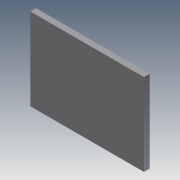
# Autodesk Inventor part: backbase
Saved by Autodesk Inventor 2011 (Build 150239000, 239)
## iProperties
Created: 2011-12-10
Part Number: backbase
Document SubType Name: Modeling
Designer: Matthew
Density: 1 g/cm^3
Author: Matthew
Autodesk Inventor part; units mm, degrees
ref_plane "YZ Plane" through (0, 0, 0) normal (1, 0, 0) x (0, 1, 0)
ref_plane "XZ Plane" through (0, 0, 0) normal (0, 1, 0) x (-1, 0, 0)
ref_plane "XY Plane" through (0, 0, 0) normal (0, 0, 1) x (1, 0, 0)
sketch "Sketch1" plane through (0, 0, 0) normal (0, 0, 1) x (1, 0, 0)
  line L0 (-30.3426, 15.2936) -> (25.6574, 15.2936)
  line L1 (25.6574, 15.2936) -> (25.6574, -29.7064)
  line L2 (25.6574, -29.7064) -> (-30.3426, -29.7064)
  line L3 (-30.3426, -29.7064) -> (-30.3426, 15.2936)
  point P0 (0, 0)
  dimension "d0" = 56
  dimension "d1" = 45
  constraints: 8 end point, 2 parallel, 1 horizontal, 1 perpendicular
  measures "d0" distance of L1.end L2.end
  measures "d1" distance of L0.end L1.end
extrude "Extrusion1" add sketch "Sketch1" along normal blind 3.175
sketch "Sketch2" plane through (25.6574, -29.7064, 0) normal (1, 0, 0) x (0, 0, -1)
  line L0 (-3.175, 45) -> (-3.175, 0) projected
  line L1 (0, 0) -> (-3.175, 0) projected
  line L2 (0, 45) -> (0, 0) projected
  line L3 (0, 45) -> (-3.175, 45) projected
  point P0 (0, 29.7064)
extrude "Extrusion2" add sketch "Sketch2" along normal blind 6.35
body "Solid1"
